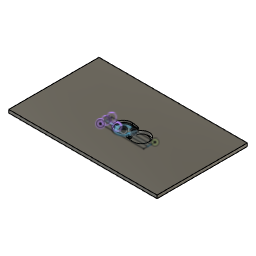
2020_09_27_ShopCoin From Wood Leftover v4 (Autodesk Fusion 360 design; units mm, degrees)
Autodesk Fusion 360 part; units mm, degrees
note: some values were not read from the file. Chosen so that the rebuilt part matches the saved one: which bodies a step acts on. Set by a fixed rule: which sketch regions a step uses.
sketch "ShopCoin" plane through (0, 0, 0) normal (0, 0, 1) x (1, 0, 0)
  line L0 (0, 10.5) -> (20, 10.5)
  circle A0 centre (32, 10.5) radius 12
  circle A1 centre (44.0302, 18) radius 1.5
  circle A2 centre (44.0302, 18) radius 3
  line L1 (20, 10.5) -> (43.3698, 6.6624) construction
  line L2 (46.8727, 17.0406) -> (43.3698, 6.6624)
  circle A3 centre (32, 10.5) radius 10
  line L3 (32, 10.5) -> (44.0302, 18) construction
  line L4 (40.486, 15.7904) -> (23.514, 15.7904)
  line L5 (23.514, 15.7904) -> (23.514, 5.2096)
  line L6 (23.514, 5.2096) -> (40.486, 5.2096)
  line L7 (40.486, 5.2096) -> (40.486, 15.7904)
  line L8 (40.486, 15.7904) -> (23.514, 5.2096) construction
  line L9 (23.514, 15.7904) -> (40.486, 5.2096) construction
  line L10 (44.4202, 20.9746) -> (33.5597, 22.3982)
  point P0 (32, 10.5)
  dimension "d5" = 20
  dimension "d6" = 24
  dimension "d9" = 1.5
  dimension "d10" = 3
  dimension "d11" = -2
  constraint coincident L0.end A0
  constraint coincident A0 L1.end
  constraint coincident A2 L2.start
  constraint tangent A2 L2
  constraint tangent A0 L2
  constraint coincident P0 A0.centre
  constraint coincident A1.centre A2.centre
  constraint horizontal L4
  constraint perpendicular L4 L5
  constraint parallel L4 L6
  constraint parallel L5 L7
  constraint coincident L3 L4.start
  constraint coincident A3 L4.start
  constraint coincident L8 P0
  constraint coincident L9 P0
  constraint coincident A2 L10.start
  constraint coincident A0 L10.end
  constraint tangent A2 L10
  constraint tangent A0 L10
  measures "d5" distance of L0.start L0.end
  measures "d6" diameter of A0
  measures "d9" distance of A1
  measures "d10" diameter of A1
sketch "WoodStick" plane through (0, 0, 0) normal (0, 0, 1) x (1, 0, 0)
  line L0 (0, 0) -> (80, 0)
  line L1 (80, 0) -> (80, 21)
  line L2 (80, 21) -> (0, 21)
  line L3 (0, 21) -> (0, 0)
  point P0 (80, 21)
  constraint horizontal L0
  constraint vertical L1
  constraint horizontal L2
  constraint vertical L3
  constraint coincident P0 L1.end
  constraint coincident L0.start L3.end
extrude "Extrude1" add sketch "WoodStick" along normal blind 5.7 makes body 1
extrude "Extrude2" add sketch "ShopCoin" along normal blind 2.2 separate body contours A0 A2 | A0 A2 L10 | A0 A2 | A0 A2 | A0 A2 L2 | A3 L7 | A3 L4 | L4 L5 L6 L7 | A3 L6 | A3 L5 makes body 2
sketch "ShopCoinBorder" plane through (0, 0, 2.2) normal (0, 0, 1) x (-1, 0, 0)
  circle A0 centre (-44.0302, -18) radius 1.5
  arc A1 (-46.8727, -17.0406) -> (-44.4202, -20.9746) centre (-44.0302, -18) ccw
  line L0 (-44.4202, -20.9746) -> (-33.5597, -22.3982)
  arc A2 (-33.5597, -22.3982) -> (-43.3698, -6.6624) centre (-32, -10.5) ccw
  line L1 (-43.3698, -6.6624) -> (-46.8727, -17.0406)
  line L2 (-46.2123, -5.703) -> (-49.7151, -16.0812)
  arc A3 (-49.7151, -16.0812) -> (-44.8101, -23.9491) centre (-44.0302, -18) ccw
  line L3 (-44.8101, -23.9491) -> (-33.9496, -25.3728)
  arc A4 (-33.9496, -25.3728) -> (-46.2123, -5.703) centre (-32, -10.5) ccw
  dimension "d19" = 3
extrude "Extrude3" add sketch "ShopCoinBorder" along normal blind 5.7 and the other way blind 5.7 separate body contours L2 A3 L3 A4 makes body 3
extrude "Extrude7" cut sketch "ShopCoin" along normal blind 5.7 and the other way blind 5.7 contours A1 bodies 1
extrude "Extrude8" cut sketch "ShopCoinBorder" along normal blind 5.7 contours A1 L0 A2 L1 bodies 1
combine "Combine1" operation cut target body 1 tool bodies 3 makes body 4 at (69.905, 12.3604, 0) makes body 5 at (5.6791, 10.1478, 0)
sketch "Sketch4" plane through (0, 0, 0) normal (0, 0, 1) x (1, 0, 0)
  line L0 (0, 7.5) -> (0, 13.5)
  line L1 (0, 13.5) -> (80, 13.5)
  line L2 (80, 13.5) -> (80, 7.5)
  line L3 (80, 7.5) -> (0, 7.5)
  line L4 (0, 21) -> (0, 0)
  line L5 (0, 10.5) -> (20, 10.5)
  dimension "d28" = 3
  dimension "d29" = 3
  constraint perpendicular L0 L1
  constraint parallel L0 L2
  constraint parallel L1 L3
  constraint coincident L0.end L4
  constraint perpendicular L0 L5
  measures "d28" distance of L1 L5
  measures "d29" distance of L3 L5
extrude "Extrude9" add sketch "ShopCoinBorder" along normal blind 3.5 separate body contours A0 | A1 L0 A2 L1 | L2 A3 L3 A4 makes body 6
extrude "Extrude10" add sketch "ShopCoin" along normal blind 2.2 contours A1 bodies 6
extrude "Extrude11" add sketch "ShopCoinBorder" against normal blind 2.2 contours L2 A3 L3 A4 bodies 6
copy_body "CopyPasteBodies2" bodies 6 makes body 7
move_body "Move3" bodies 7 to x (-1, 0, 0) y (0, -1, 0) z (0, 0, 1) at (88.0605, 36, 0)
move_body "Move4" bodies 7 to x (1, 0, 0) y (0, 1, 0) z (0, 0, 1) at (8.6234, -14.9661, 0)
sketch "Sketch5" plane through (0, 0, 0) normal (0, 0, 1) x (1, 0, 0)
  line L0 (-101.959, -67.5979) -> (172.2674, -67.5979)
  line L1 (172.2674, -67.5979) -> (172.2674, 99.2567)
  line L2 (172.2674, 99.2567) -> (-101.959, 99.2567)
  line L3 (-101.959, 99.2567) -> (-101.959, -67.5979)
  constraint horizontal L0
  constraint vertical L1
  constraint horizontal L2
  constraint vertical L3
extrude "Extrude12" add sketch "Sketch5" along normal blind 5.7 separate body makes body 8
combine "Combine2" operation cut target body 8 tool bodies 6 7 keep tools makes body 9 at (58.398, 11.3248, 2.2) makes body 10 at (-62.2819, 14.5434, 0)
delete_body "RemoveBody2" bodies 4
delete_body "RemoveBody3" bodies 5
hidden bodies 1 6 7
equation "d13 = WoodHeight"
equation "d15 = CoinHeight"
equation "WoodHeight = 5.7 mm"
equation "CoinHeight = 2.2 mm"
equation "d20 = WoodHeight"
equation "d22 = WoodHeight"
equation "TabHeight = 0.3 mm"
equation "d39 = WoodHeight"
equation "d41 = WoodHeight"
equation "d43 = WoodHeight"
equation "d45 = WoodHeight - CoinHeight"
equation "d47 = CoinHeight"
equation "d49 = -CoinHeight"
equation "d52 = WoodHeight"
named bodies: "WoodPart", "Original CoinShape", "WoodPart (2)", "WoodPart (4)", "CoinShapePattern 1", "CoinShapePattern", "CoinShapePattern 2", "Produced CoinShape 1", "Produced CoinShape 2", "Wood"
